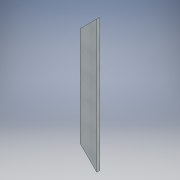
# Autodesk Inventor part: Fata_3
Saved by Autodesk Inventor 2017 (Build 210142000, 142)
## iProperties
Created: 2017-06-02
Part Number: Fata_3
Material: Generic
Document SubType Name: Modeling
Designer: crush
Density: 1 g/cm^3
Appearance: Wood - Painted White
Author: crush
Autodesk Inventor part; units mm, degrees
ref_plane "YZ Plane" through (0, 0, 0) normal (1, 0, 0) x (0, 1, 0)
ref_plane "XZ Plane" through (0, 0, 0) normal (0, 1, 0) x (-1, 0, 0)
ref_plane "XY Plane" through (0, 0, 0) normal (0, 0, 1) x (1, 0, 0)
sketch "Sketch1" plane through (0, 0, 0) normal (0, 1, 0) x (-1, 0, 0)
  line L0 (0, 0) -> (0, -600)
  line L1 (0, 0) -> (-100, 0)
  line L2 (-100, 0) -> (-100, 100)
  line L3 (-100, 100) -> (0, 0)
  line L4 (0, -600) -> (-100, -600)
  line L5 (-100, -600) -> (-100, -700)
  line L6 (-100, -700) -> (0, -600)
  line L7 (-100, -600) -> (-100, 0)
  dimension "d0" = 600
  dimension "d1" = 100
  dimension "d2" = 100
  dimension "d3" = 100
  dimension "d4" = 100
  constraints: 16 end point, 2 horizontal, 2 perpendicular, 2 vertical
  measures "d0" distance of L0.start L0.end
  measures "d1" distance of L0.start L1.end
  measures "d2" distance of L1.end L2.end
  measures "d3" distance of L0.end L4.end
  measures "d4" distance of L4.end L5.end
extrude "Extrusion1" add sketch "Sketch1" along normal blind 18
body "Solid1"
